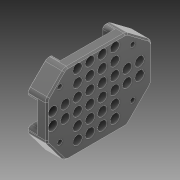
# Autodesk Inventor part: 0.25in From Edge Box Tube Drill Guide
Saved by Autodesk Inventor 2022 (Build 260153000, 153)
## iProperties
Created: 2022-01-31
Part Number: 0.25in From Edge Box Tube Drill Guide
Material: Nylon 6/6
Document SubType Name: Modeling
Designer: Desktop
Density: 1.13 g/cm^3
Appearance: Smooth - Black
Author: Desktop
Autodesk Inventor part; units mm, degrees
ref_plane "YZ Plane" through (0, 0, 0) normal (1, 0, 0) x (0, 1, 0)
ref_plane "XZ Plane" through (0, 0, 0) normal (0, 1, 0) x (-1, 0, 0)
sketch "Sketch1" plane through (0, 0, 0) normal (1, 0, 0) x (0, 1, 0)
  line L0 (31.75, 19.05) -> (-31.75, 19.05) construction
  line L1 (-31.75, 19.05) -> (-31.75, -19.05) construction
  line L2 (-31.75, -19.05) -> (31.75, -19.05) construction
  line L3 (31.75, -19.05) -> (31.75, 19.05) construction
  circle A0 centre (31.75, 19.05) radius 2.4892
  circle A1 centre (31.75, 6.35) radius 2.4892
  circle A2 centre (31.75, -6.35) radius 2.4892
  circle A3 centre (31.75, -19.05) radius 2.4892
  circle A4 centre (19.05, 19.05) radius 2.4892
  circle A5 centre (19.05, 6.35) radius 2.4892
  circle A6 centre (19.05, -6.35) radius 2.4892
  circle A7 centre (19.05, -19.05) radius 2.4892
  circle A8 centre (6.35, 19.05) radius 2.4892
  circle A9 centre (6.35, 6.35) radius 2.4892
  circle A10 centre (6.35, -6.35) radius 2.4892
  circle A11 centre (6.35, -19.05) radius 2.4892
  circle A12 centre (-6.35, 19.05) radius 2.4892
  circle A13 centre (-6.35, 6.35) radius 2.4892
  circle A14 centre (-6.35, -6.35) radius 2.4892
  circle A15 centre (-6.35, -19.05) radius 2.4892
  line L4 (31.75, 19.05) -> (-31.75, -19.05) construction
  line L5 (31.75, -19.05) -> (-31.75, 19.05) construction
  line L6 (38.1, 25.4) -> (-38.1, 25.4)
  line L7 (-38.1, 25.4) -> (-38.1, -25.4) construction
  line L8 (-38.1, -25.4) -> (38.1, -25.4)
  line L9 (38.1, -25.4) -> (38.1, 25.4)
  line L10 (-38.1, 25.4) -> (-44.45, 25.4)
  line L11 (-44.45, 31.75) -> (-44.45, -25.4)
  line L12 (-44.45, -25.4) -> (-38.1, -25.4)
  line L13 (-38.1, -25.4) -> (-38.1, 25.4) construction
  line L14 (38.1, 31.75) -> (38.1, 25.4)
  line L15 (38.1, -25.4) -> (-44.45, -25.4)
  line L16 (-44.45, -25.4) -> (-44.45, -31.75)
  line L17 (38.1, -31.75) -> (38.1, -25.4)
  line L18 (0, 0) -> (33.1324, 0) construction
  line L19 (19.05, 50.8) -> (-19.05, 50.8)
  line L20 (-12.7, -50.8) -> (-12.7, -57.15) construction
  line L21 (-19.05, -57.15) -> (19.05, -57.15)
  line L22 (0, 0) -> (0, -7.8291) construction
  circle A16 centre (-19.05, 19.05) radius 2.4892
  circle A17 centre (-19.05, 6.35) radius 2.4892
  circle A18 centre (-19.05, -6.35) radius 2.4892
  circle A19 centre (-19.05, -19.05) radius 2.4892
  circle A20 centre (-31.75, 19.05) radius 2.4892
  circle A21 centre (-31.75, 6.35) radius 2.4892
  circle A22 centre (-31.75, -6.35) radius 2.4892
  circle A23 centre (-31.75, -19.05) radius 2.4892
  circle A24 centre (6.35, 31.75) radius 2.4892
  circle A25 centre (-6.35, 31.75) radius 2.4892
  circle A26 centre (6.35, 44.45) radius 2.4892
  circle A27 centre (-6.35, 44.45) radius 2.4892
  circle A28 centre (6.35, -31.75) radius 2.4892
  circle A29 centre (-6.35, -31.75) radius 2.4892
  circle A30 centre (6.35, -44.45) radius 2.4892
  circle A31 centre (-6.35, -44.45) radius 2.4892
  line L23 (-44.45, 31.75) -> (-19.05, 50.8)
  line L24 (38.1, 31.75) -> (19.05, 50.8)
  line L25 (-44.45, -31.75) -> (-19.05, -57.15)
  line L26 (38.1, -31.75) -> (19.05, -57.15)
  line L27 (12.7, 57.15) -> (-12.7, 57.15)
  line L28 (-12.7, 57.15) -> (-12.7, -57.15)
  line L29 (-12.7, -57.15) -> (12.7, -57.15)
  line L30 (12.7, -57.15) -> (12.7, 57.15)
  line L31 (12.7, 57.15) -> (-12.7, -57.15) construction
  line L32 (-12.7, 57.15) -> (12.7, -57.15) construction
  point P0 (12.7, -57.15)
  point P1 (0, 50.8)
  point P2 (-12.7, 25.4)
  point P3 (-12.7, -25.4)
  point P4 (-12.7, -25.4)
  dimension "d0" = 4.9784
  dimension "d5" = 12.7
  dimension "d8" = 12.7
  dimension "d11" = 50.8
  dimension "d12" = 6.35
  dimension "d13" = 6.35
  dimension "d32" = 12.7
  dimension "d37" = 6.35
  dimension "d38" = 12.7
  dimension "d47" = 12.7
  dimension "d50" = 25.4
  constraints: 66 end point, 32 centre point, 10 parallel, 7 horizontal, 6 perpendicular, 4 midpoint, 4 point on line, 4 symmetric about line, 4 vertical, 3 coincident, 3 vertical alignment, 2 collinear, 2 equal length, 1 horizontal alignment, 61 other
  measures "d0" diameter of A0
  measures "d5" distance of L4.start A1.centre
  measures "d8" distance of L4.start A4.centre
  measures "d11" distance between parallel lines of L8 L6
  measures "d12" distance between parallel lines of L7 L11
  measures "d13" distance of L14.start L6.start
  measures "d32" distance of A8.centre A24.centre
  measures "d37" distance from line of A26.centre L19
  measures "d38" distance from line of L21 A30.centre
  measures "d47" horizontal distance of A27.centre L19.end
  measures "d50" distance between parallel lines of L30 L28
extrude "Extrusion2" add sketch "Sketch1" along normal blind 9.525 contours L9 L8 L30 L6 | L6 L30 L19 L24 L14 | L30 L8 L28 L6 | L6 L28 L19 L30 | L17 L26 L21 L30 L8 | L28 L8 L12 L11 L10 L6 | L6 L10 L11 L23 L19 L28 | L30 L21 L28 L8 | L28 L21 L25 L16 L12 L8
sketch "Sketch2" plane through (0, 0, 0) normal (-1, 0, 0) x (0, 0, 1)
  line L0 (31.75, -44.45) -> (-31.75, -44.45) projected
  line L1 (50.8, -19.05) -> (31.75, -44.45) projected
  line L2 (50.8, 19.05) -> (50.8, -19.05) projected
  line L3 (31.75, 38.1) -> (50.8, 19.05) projected
  line L4 (-31.75, 38.1) -> (31.75, 38.1) projected
  line L5 (-57.15, 19.05) -> (-31.75, 38.1) projected
  line L6 (-57.15, -19.05) -> (-57.15, 19.05) projected
  line L7 (-31.75, -44.45) -> (-57.15, -19.05) projected
  circle A0 centre (-19.05, -6.35) radius 2.4892 projected
  circle A1 centre (6.35, -6.35) radius 2.4892 projected
  circle A2 centre (-19.05, 6.35) radius 2.4892 projected
  circle A3 centre (6.35, 6.35) radius 2.4892 projected
  circle A4 centre (19.05, 6.35) radius 2.4892 projected
  circle A5 centre (-6.35, 6.35) radius 2.4892 projected
  circle A6 centre (19.05, -6.35) radius 2.4892 projected
  circle A7 centre (-6.35, -6.35) radius 2.4892 projected
  circle A8 centre (-6.35, -19.05) radius 2.4892 projected
  circle A9 centre (44.45, -6.35) radius 2.4892 projected
  circle A10 centre (44.45, 6.35) radius 2.4892 projected
  circle A11 centre (-19.05, -31.75) radius 2.4892 projected
  circle A12 centre (-6.35, -31.75) radius 2.4892 projected
  circle A13 centre (6.35, -31.75) radius 2.4892 projected
  circle A14 centre (19.05, -31.75) radius 2.4892 projected
  circle A15 centre (6.35, 19.05) radius 2.4892 projected
  circle A16 centre (19.05, 19.05) radius 2.4892 projected
  circle A17 centre (19.05, 31.75) radius 2.4892 projected
  circle A18 centre (6.35, 31.75) radius 2.4892 projected
  circle A19 centre (-6.35, 31.75) radius 2.4892 projected
  circle A20 centre (-19.05, 31.75) radius 2.4892 projected
  circle A21 centre (-6.35, 19.05) radius 2.4892 projected
  circle A22 centre (-19.05, 19.05) radius 2.4892 projected
  circle A23 centre (31.75, 6.35) radius 2.4892 projected
  circle A24 centre (31.75, -6.35) radius 2.4892 projected
  circle A25 centre (6.35, -19.05) radius 2.4892 projected
  circle A26 centre (19.05, -19.05) radius 2.4892 projected
  circle A27 centre (-19.05, -19.05) radius 2.4892 projected
  circle A28 centre (-31.75, 6.35) radius 2.4892 projected
  circle A29 centre (-44.45, -6.35) radius 2.4892 projected
  circle A30 centre (-44.45, 6.35) radius 2.4892 projected
  circle A31 centre (-31.75, -6.35) radius 2.4892 projected
  line L8 (-25.4, -44.45) -> (25.4, -44.45)
  line L9 (25.4, -44.45) -> (25.4, 44.45)
  line L10 (25.4, 44.45) -> (-25.4, 44.45)
  line L11 (-25.4, 44.45) -> (-25.4, -44.45)
  line L12 (-25.4, -44.45) -> (25.4, 44.45) construction
  line L13 (25.4, -44.45) -> (-25.4, 44.45) construction
  line L14 (-57.15, -12.7) -> (57.15, -12.7)
  line L15 (57.15, -12.7) -> (57.15, 12.7)
  line L16 (57.15, 12.7) -> (-57.15, 12.7)
  line L17 (-57.15, 12.7) -> (-57.15, -12.7)
  line L18 (-57.15, -12.7) -> (57.15, 12.7) construction
  line L19 (57.15, -12.7) -> (-57.15, 12.7) construction
  line L20 (31.75, -44.45) -> (-31.75, -44.45) projected
  line L21 (-57.15, -19.05) -> (-57.15, 19.05) projected
  line L22 (63.5, -19.05) -> (-63.5, -19.05)
  line L23 (-63.5, -19.05) -> (-63.5, 19.05)
  line L24 (-63.5, 19.05) -> (63.5, 19.05)
  line L25 (63.5, 19.05) -> (63.5, -19.05)
  line L26 (31.75, 50.8) -> (31.75, -50.8)
  line L27 (31.75, -50.8) -> (-31.75, -50.8)
  line L28 (-31.75, -50.8) -> (-31.75, 50.8)
  line L29 (-31.75, 50.8) -> (31.75, 50.8)
  circle A32 centre (-37.3296, -24.6296) radius 5.5796 construction
  circle A33 centre (-37.3296, 24.6296) radius 5.5796 construction
  circle A34 centre (37.3296, 24.6296) radius 5.5796 construction
  circle A35 centre (37.3296, -24.6296) radius 5.5796 construction
  circle A36 centre (37.3296, 24.6296) radius 2.4892
  circle A37 centre (-37.3296, 24.6296) radius 2.4892
  circle A38 centre (-37.3296, -24.6296) radius 2.4892
  circle A39 centre (37.3296, -24.6296) radius 2.4892
  point P0 (0, 0)
  point P1 (25.4, 38.1)
  point P2 (25.4, 12.7)
  point P3 (50.8, 12.7)
  point P4 (-25.4, 12.7)
  point P5 (-25.4, 38.1)
  point P6 (-25.4, -12.7)
  point P7 (50.8, -12.7)
  point P8 (25.4, -12.7)
  dimension "d51" = 50.8
  dimension "d52" = 25.4
  dimension "d53" = 6.35
  dimension "d54" = 6.35
  dimension "d59" = 4.9784
  constraints: 40 end point, 9 tangent, 8 centre point, 8 parallel, 6 equal radius, 4 midpoint, 4 perpendicular, 2 horizontal, 2 point on line, 6 other
  measures "d51" distance of L10.end L9.end
  measures "d52" distance of L15.end L14.end
  measures "d53" distance between parallel lines of L14 L22
  measures "d54" distance between parallel lines of L9 L26
  measures "d59" diameter of A36
extrude "Extrusion3" add sketch "Sketch2" along normal blind 9.525 contours L26 L22 L1 | L0 L9 L22 L26 | L22 L26 L14 L2 | L22 L9 L14 L26 | L0 L28 L22 L11 | L7 L22 L28 | L22 L28 L14 L11 | L16 L26 L24 L2 | L6 L14 L28 L22 | L9 L24 L26 L16 | L24 L26 L3 | L16 L28 L24 L11 | L9 L4 L26 L24 | L6 L24 L28 L16 | L24 L28 L4 L11 | L5 L28 L24 | A36 | A37 | A38 | A39
fillet "Fillet3" radius 3.175 4 edges at (-4.7625, -12.7, -25.4) (-4.7625, -12.7, 25.4) (-4.7625, 12.7, 25.4) (-4.7625, 12.7, -25.4)
extrude "Extrusion4" cut sketch "Sketch2" along normal through all both and the other way through all contours A36 | A37 | A38 | A39
fillet "Fillet4" radius 6.35 8 edges at (0, 38.1, -31.75) (0, 38.1, 31.75) (0, 19.05, 50.8) (0, -19.05, 50.8) (0, -44.45, 31.75) (0, -44.45, -31.75) (0, -19.05, -57.15) (0, 19.05, -57.15)
sketch "Sketch3" plane through (0, 0, 0) normal (-1, 0, 0) x (0, 0, 1)
  circle A0 centre (19.05, -31.75) radius 2.4892 projected
  circle A1 centre (6.35, -31.75) radius 2.4892 projected
  circle A2 centre (-6.35, -31.75) radius 2.4892 projected
  circle A3 centre (-19.05, -31.75) radius 2.4892 projected
  circle A4 centre (19.05, -19.05) radius 2.4892 projected
  circle A5 centre (6.35, -19.05) radius 2.4892 projected
  circle A6 centre (-6.35, -19.05) radius 2.4892 projected
  circle A7 centre (-19.05, -19.05) radius 2.4892 projected
  circle A8 centre (44.45, -6.35) radius 2.4892 projected
  circle A9 centre (31.75, -6.35) radius 2.4892 projected
  circle A10 centre (31.75, 6.35) radius 2.4892 projected
  circle A11 centre (44.45, 6.35) radius 2.4892 projected
  circle A12 centre (19.05, -6.35) radius 2.4892 projected
  circle A13 centre (6.35, -6.35) radius 2.4892 projected
  circle A14 centre (-6.35, -6.35) radius 2.4892 projected
  circle A15 centre (-19.05, -6.35) radius 2.4892 projected
  circle A16 centre (-31.75, -6.35) radius 2.4892 projected
  circle A17 centre (-44.45, -6.35) radius 2.4892 projected
  circle A18 centre (19.05, 6.35) radius 2.4892 projected
  circle A19 centre (6.35, 6.35) radius 2.4892 projected
  circle A20 centre (-6.35, 6.35) radius 2.4892 projected
  circle A21 centre (-19.05, 6.35) radius 2.4892 projected
  circle A22 centre (-44.45, 6.35) radius 2.4892 projected
  circle A23 centre (-31.75, 6.35) radius 2.4892 projected
  circle A24 centre (19.05, 19.05) radius 2.4892 projected
  circle A25 centre (6.35, 19.05) radius 2.4892 projected
  circle A26 centre (-6.35, 19.05) radius 2.4892 projected
  circle A27 centre (-19.05, 19.05) radius 2.4892 projected
  circle A28 centre (19.05, 31.75) radius 2.4892 projected
  circle A29 centre (6.35, 31.75) radius 2.4892 projected
  circle A30 centre (-6.35, 31.75) radius 2.4892 projected
  circle A31 centre (-19.05, 31.75) radius 2.4892 projected
  point P0 (0, 0)
  point P1 (-6.35, 6.35)
  constraints: 32 coincident
hole "Hole1" at (0, -31.75, 19.05) at (0, -31.75, 6.35) at (0, -31.75, -6.35) at (0, -31.75, -19.05) at (0, -19.05, 19.05) at (0, -19.05, 6.35) at (0, -19.05, -6.35) at (0, -19.05, -19.05) at (0, -6.35, 44.45) at (0, -6.35, 31.75) at (0, 6.35, 31.75) at (0, 6.35, 44.45) at (0, -6.35, 19.05) at (0, -6.35, 6.35) at (0, -6.35, -6.35) at (0, -6.35, -19.05) at (0, -6.35, -31.75) at (0, -6.35, -44.45) at (0, 6.35, 19.05) at (0, 6.35, 6.35) at (0, 6.35, -6.35) at (0, 6.35, -19.05) at (0, 6.35, -44.45) at (0, 6.35, -31.75) at (0, 19.05, 19.05) at (0, 19.05, 6.35) at (0, 19.05, -6.35) at (0, 19.05, -19.05) at (0, 31.75, 19.05) at (0, 31.75, 6.35) at (0, 31.75, -6.35) at (0, 31.75, -19.05) direction (1, 0, 0) diameter 9.4742 depth 9.525 tip angle 118 counterbore diameter 12.065 counterbore depth 1.524
chamfer "Chamfer2" distance 1.5875 angle 45 16 edges at (9.525, -43.7796, 31.4148) (9.525, -31.3267, 41.5925) (9.525, -18.9414, 50.4741) (9.525, -0.2568, 50.8) (9.525, 18.8498, 50.3166) (9.525, 28.575, 41.275) (9.525, 37.6166, 31.5498) (9.525, 38.1, -0.2568) (9.525, 37.7741, -31.6414) (9.525, 28.8925, -44.0267) (9.525, 18.7148, -56.4796) (9.525, -0.2724, -57.15) (9.525, -18.8498, -56.6666) (9.525, -31.75, -44.45) (9.525, -43.9666, -31.5498) (9.525, -44.45, -0.2724)
fillet "Fillet5" radius 3.175 8 edges at (-4.7625, -12.7, 50.8) (-4.7625, 12.7, 50.8) (-4.7625, 38.1, -25.4) (-4.7625, 38.1, 25.4) (-4.7625, -44.45, -25.4) (-4.7625, -12.7, -57.15) (-4.7625, 12.7, -57.15) (-4.7625, -44.45, 25.4)
chamfer "Chamfer3" distance 0.3969 angle 45 39 edges at (-9.525, -31.75, -44.45) (-9.525, -43.9666, -31.5498) (-9.525, -44.45, -28.8471) (-9.525, -44.45, 28.5748) (-9.525, -43.5202, -26.3298) (-9.525, -28.5752, -25.4) (-9.525, -13.6299, -26.3299) (-9.525, -12.7, -41.2752) (-9.525, -13.6298, -56.2202) (-9.525, -16.1471, -57.15) (-9.525, -18.8498, -56.6666) (-9.525, 12.7, -41.2752) (-9.525, 13.6299, -26.3299) (-9.525, 25.4002, -25.4) (-9.525, 37.1702, -26.3298) (-9.525, 38.1, -29.1039) (-9.525, 38.1, 28.8471) (-9.525, 37.7741, -31.6414) (-9.525, 28.8925, -44.0267) (-9.525, 18.7148, -56.4796) (-9.525, 13.6298, -56.2202) (-9.525, 12.7, 38.1003) (-9.525, 13.6298, 49.8702) (-9.525, 16.1471, 50.8) (-9.525, 18.8498, 50.3166) (-9.525, 28.575, 41.275) (-9.525, 37.6166, 31.5498) (-9.525, 37.1702, 26.3298) (-9.525, 25.4002, 25.4) (-9.525, 13.6299, 26.3299) (-9.525, -12.7, 38.1003) (-9.525, -13.6299, 26.3299) (-9.525, -28.5752, 25.4) (-9.525, -43.5202, 26.3298) (-9.525, -43.7796, 31.4148) (-9.525, -31.3267, 41.5925) (-9.525, -18.9414, 50.4741) (-9.525, -16.4039, 50.8) (-9.525, -13.6298, 49.8702)
ref_plane "Work Plane1" through (-12.7, 0, 0) normal (-1, 0, 0) x (0, 0, 1)
body "Solid1"
body "Solid2"
